Autodesk Inventor part; units mm, degrees
(part 2 of 2)
  spline S9 degree 3 poles (2.586, 0.2698) (2.5854, 0.2691) (2.5801, 0.2629) (2.5701, 0.2513) (2.5558, 0.2352) (2.5415, 0.2194) (2.5273, 0.204) (2.513, 0.1891) (2.4988, 0.1744) (2.4845, 0.1602) (2.4704, 0.1464) (2.4562, 0.1329) (2.4421, 0.1197) (2.428, 0.107) (2.414, 0.0946) (2.4001, 0.0825) (2.3862, 0.0708) (2.3724, 0.0595) (2.3586, 0.0485) (2.345, 0.0378) (2.3315, 0.0275) (2.318, 0.0175) (2.3047, 0.0078) (2.2915, -0.0015) (2.2784, -0.0105) (2.2654, -0.0192) (2.2525, -0.0276) (2.2398, -0.0356) (2.2273, -0.0434) (2.2148, -0.0509) (2.2026, -0.058) (2.1905, -0.0649) (2.1785, -0.0715) (2.1667, -0.0778) (2.1551, -0.0839) (2.1437, -0.0896) (2.1325, -0.0951) (2.1214, -0.1004) (2.1105, -0.1054) (2.0999, -0.1101) (2.0894, -0.1147) (2.0791, -0.1189) (2.0691, -0.123) (2.0592, -0.1268) (2.0496, -0.1304) (2.0402, -0.1338) (2.031, -0.1369) (2.0221, -0.1399) (2.0134, -0.1427) (2.0049, -0.1453) (1.9967, -0.1477) (1.9887, -0.1499) (1.9809, -0.152) (1.9734, -0.1539) (1.9662, -0.1556) (1.9592, -0.1572) (1.9524, -0.1586) (1.9459, -0.1599) (1.9397, -0.1611) (1.9338, -0.1622) (1.9281, -0.1631) (1.9226, -0.1639) (1.9175, -0.1646) (1.9126, -0.1652) (1.908, -0.1658) (1.9036, -0.1662) (1.8996, -0.1666) (1.8958, -0.1668) (1.8923, -0.1671) (1.889, -0.1672) (1.8861, -0.1674) (1.8834, -0.1674) (1.881, -0.1675) (1.8789, -0.1675) (1.8771, -0.1675) (1.8694, -0.1673) (1.8573, -0.1649) (1.8404, -0.1634) (1.8249, -0.1624) (1.8097, -0.1622) (1.7946, -0.1625) (1.7796, -0.1635) (1.7648, -0.1653) (1.7499, -0.1679) (1.735, -0.1714) (1.72, -0.1759) (1.7049, -0.1818) (1.6896, -0.1891) (1.6741, -0.1983) (1.6586, -0.2097) (1.6434, -0.2238) (1.6291, -0.2408) (1.6165, -0.261) (1.6073, -0.2828) (1.6021, -0.3014) (1.5996, -0.3158) (1.5965, -0.33) (1.5942, -0.3492) (1.5944, -0.3728) (1.5984, -0.3963) (1.6051, -0.4175) (1.6138, -0.4363) (1.6238, -0.4527) (1.6347, -0.4671) (1.6461, -0.4797) (1.6579, -0.4908) (1.67, -0.5008) (1.6825, -0.5096) (1.6952, -0.5177) (1.7083, -0.525) (1.7217, -0.5316) (1.7355, -0.5376) (1.7498, -0.5432) (1.7644, -0.5481) (1.7806, -0.5532) (1.7928, -0.5556) (1.7999, -0.5584) (1.8016, -0.559) (1.8036, -0.5598) (1.8058, -0.5608) (1.8082, -0.5619) (1.8109, -0.5631) (1.8138, -0.5645) (1.817, -0.566) (1.8204, -0.5677) (1.824, -0.5696) (1.8279, -0.5717) (1.8319, -0.5739) (1.8362, -0.5763) (1.8407, -0.579) (1.8454, -0.5818) (1.8503, -0.5848) (1.8554, -0.588) (1.8608, -0.5915) (1.8663, -0.5951) (1.8719, -0.599) (1.8778, -0.6032) (1.8839, -0.6075) (1.8901, -0.6121) (1.8965, -0.617) (1.903, -0.6221) (1.9097, -0.6274) (1.9166, -0.6331) (1.9236, -0.6389) (1.9307, -0.6451) (1.938, -0.6515) (1.9454, -0.6582) (1.953, -0.6652) (1.9606, -0.6725) (1.9684, -0.68) (1.9762, -0.6879) (1.9842, -0.696) (1.9923, -0.7045) (2.0004, -0.7132) (2.0087, -0.7223) (2.017, -0.7316) (2.0253, -0.7413) (2.0338, -0.7513) (2.0423, -0.7616) (2.0508, -0.7723) (2.0594, -0.7833) (2.068, -0.7946) (2.0767, -0.8062) (2.0854, -0.8181) (2.0941, -0.8304) (2.1028, -0.8431) (2.1115, -0.856) (2.1202, -0.8693) (2.1288, -0.883) (2.1375, -0.897) (2.1462, -0.9113) (2.1548, -0.926) (2.1633, -0.9411) (2.1718, -0.9565) (2.1803, -0.9722) (2.1887, -0.9883) (2.197, -1.0047) (2.2053, -1.0215) (2.2134, -1.0387) (2.2215, -1.0562) (2.2295, -1.0741) (2.2373, -1.0923) (2.2451, -1.1108) (2.2527, -1.1298) (2.2602, -1.1491) (2.2675, -1.1687) (2.2747, -1.1887) (2.2821, -1.2099) (2.2869, -1.2244) (2.2895, -1.2322) knots 0.016719 0.016719 0.016719 0.016719 0.017808 0.026543 0.035166 0.043676 0.052073 0.060357 0.068528 0.076587 0.084533 0.092367 0.100087 0.107695 0.115191 0.122573 0.129843 0.137 0.144045 0.150977 0.157796 0.164502 0.171095 0.177576 0.183945 0.1902 0.196343 0.202373 0.20829 0.214095 0.219787 0.225366 0.230832 0.236186 0.241427 0.246556 0.251571 0.256474 0.261264 0.265942 0.270507 0.274959 0.279298 0.283525 0.287639 0.29164 0.295528 0.299304 0.302967 0.306518 0.309956 0.31328 0.316493 0.319592 0.322579 0.325453 0.328215 0.330863 0.333399 0.335823 0.338133 0.340331 0.342416 0.344389 0.346248 0.347996 0.34963 0.351151 0.35256 0.353856 0.35504 0.356111 0.357069 0.357914 0.358647 0.359267 0.367127 0.373439 0.379636 0.385738 0.391769 0.397757 0.403738 0.409752 0.415852 0.422098 0.428563 0.435333 0.442503 0.450171 0.458425 0.467319 0.476841 0.486882 0.495598 0.5 0.504402 0.513118 0.523159 0.532681 0.541575 0.549829 0.557497 0.564667 0.571437 0.577902 0.584148 0.590248 0.596262 0.602243 0.608231 0.614262 0.620364 0.626561 0.632873 0.640733 0.641353 0.642086 0.642931 0.643889 0.64496 0.646144 0.64744 0.648849 0.65037 0.652004 0.653752 0.655611 0.657584 0.659669 0.661867 0.664177 0.666601 0.669137 0.671785 0.674547 0.677421 0.680408 0.683507 0.68672 0.690044 0.693482 0.697033 0.700696 0.704472 0.70836 0.712361 0.716475 0.720702 0.725041 0.729493 0.734058 0.738736 0.743526 0.748429 0.753444 0.758573 0.763814 0.769168 0.774634 0.780213 0.785905 0.79171 0.797627 0.803657 0.8098 0.816055 0.822424 0.828905 0.835498 0.842204 0.849023 0.855955 0.863 0.870157 0.877427 0.884809 0.892305 0.899913 0.907633 0.915467 0.923413 0.931472 0.939643 0.947927 0.956324 0.964834 0.973457 0.983281 0.983281 0.983281 0.983281
  arc A9 (2.586, 0.2698) -> (2.5765, 0.3488) centre (0, 0) ccw
  circle A10 centre (0, 0) radius 0.45
  constraints: 20 point on circle, 11 centre point, 20 other
extrude "Extrusion1" add sketch "Sketch1" against normal blind 2.9972
body "Solid1"
